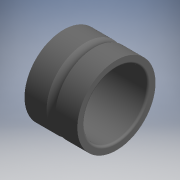
# Autodesk Inventor part: MF63ZZ Inner Ring
Saved by Autodesk Inventor 2017.3 (Build 213256000, 256)
## iProperties
Part Number: MF63ZZ Inner Ring
Material: Generic
Catalog Web Link: www.cadenas.de
Description: shielded_type_zz_zzs_IR-
Vendor: NSK_RB
Document SubType Name: Modeling
Designer: partserver
Manufacturer: NSK_RB
Mass: 0.00900788 g
Surface Area: 0.59285 cm^2
Volume: 0.00900788 cm^3
Density: 1 g/cm^3
Appearance: PSOLRGB-128-128-128
Category: PARTsolutions
Company: NSK_RB
Title: MF63ZZ Inner Ring
Author: Cadenas PARTsolutions
PSOL_IDENT_0: {$CADENAS_DATA\23d-libs\nsk_rb\roller_bearings\deep_groove_bb\exstra_small_miniatur_bb\metric_design
PSOL_IDENT_1: _with_flange\shielded_type_zz_zzs_ir_1.prj},192 {VTYP=3D},{NB=MF63ZZ Inner Ring},{LINA=MF63ZZ Inner
PSOL_IDENT_2: Ring},{NN=shielded_type_zz_zzs_IR},{DATE=10.04.2020 04:57:40},{GEOMDATE=04.01.2008 00:00:00},{VERSIO
PSOL_IDENT_3: N=},{LINEID=120},{WBVAR=},{WBNUMERIC=}  {NB=MF63ZZ Inner Ring},{LINA=MF63ZZ Inner Ring},{KT=DUMMY},{
PSOL_IDENT_4: IDNR=},{STAN=},{ORDER=MF63ZZ},{SD=3.0},{X=3.0},{D=6},{DD=6},{DD1=0.0},{D2=7.2},{DD2=7.2},{B=0.0},{B1=
PSOL_IDENT_5: 2.5},{CC1=0.0},{C2=0.6},{CC2=0.6},{R=0.00},{R1=0.10},{DI1=3.70},{DI2=3.70},{SDE1=4.90},{SDE2=5.40},{
PSOL_IDENT_6: CR1=208},{COR1=74},{CR2=21},{COR2=7.5},{LG=71000},{LO=80000},{DA=0.0},{DB=3.7},{RA=0.00},{RB=0.10},{
PSOL_IDENT_7: MASS=0.33},{SC=1},{N=12}
NB: MF63ZZ Inner Ring
NN: shielded_type_zz_zzs_IR
NBSYN: $ORDER. Inner Ring
LINA: MF63ZZ Inner Ring
CATALOG: NSK Rolling Bearing
ORDER: MF63ZZ
SD: 3
X: 3
D: 6
DD: 6
DD1: 0
D2: 7.2
DD2: 7.2
B: 0
B1: 2.5
CC1: 0
C2: 0.6
CC2: 0.6
R: 0
R1: 0.1
DI1: 3.7
DI2: 3.7
SDE1: 4.9
SDE2: 5.4
CR1: 208
COR1: 74
CR2: 21
COR2: 7.5
LG: 71000
LO: 80000
DA: 0
DB: 3.7
RA: 0
RB: 0.1
MASS: 0.33
SC: 1
SUPPLIER: NSK_RB
ARTICLENO: MF63ZZ Inner Ring
BOMINFO: MF63ZZ Inner Ring
CREATOR: CADENAS GmbH
Autodesk Inventor part; units mm, degrees
sketch "Sketch_1" plane through (0, 0, 0) normal (0, 0, 1) x (1, 0, 0)
  line L0 (2.5, 0) -> (0, 0)
  arc A0 (0, 1.6) -> (0.1, 1.5) centre (0.1, 1.6) ccw
  line L1 (0.1, 1.5) -> (2.4, 1.5)
  arc A1 (2.4, 1.5) -> (2.5, 1.6) centre (2.4, 1.6) ccw
  line L2 (2.5, 1.6) -> (2.5, 1.85)
  line L3 (2.5, 1.85) -> (1.4562, 1.85)
  arc A2 (1.0438, 1.85) -> (1.4562, 1.85) centre (1.25, 2.25) ccw
  line L4 (1.0438, 1.85) -> (0, 1.85)
  line L5 (0, 1.85) -> (0, 1.6)
  constraints: 12 end point, 6 point on circle, 3 centre point
revolve "Revolution1" add sketch "Sketch_1" angle 360 about axis through (2.5, 0, 0) along (1, 0, 0)
ref_plane "ip_st_1_1_XY" through (1.25, 2.25, 0) normal (1, 0, 0) x (0, 0, -1)
ref_plane "ip_st_1_1_YZ" through (1.25, 2.25, 0) normal (0, 0, -1) x (0, 1, 0)
ref_plane "ip_st_1_1_ZX" through (1.25, 2.25, 0) normal (0, 1, 0) x (1, 0, 0)
ref_plane "ip_st_1_10_XY" through (1.25, 0, -2.25) normal (1, 0, 0) x (0, 0, -1)
ref_plane "ip_st_1_10_YZ" through (1.25, 0, -2.25) normal (0, 0, -1) x (0, 1, 0)
ref_plane "ip_st_1_10_ZX" through (1.25, 0, -2.25) normal (0, 1, 0) x (1, 0, 0)
ref_plane "ip_st_1_11_XY" through (1.25, 1.125, -1.9486) normal (1, 0, 0) x (0, 0, -1)
ref_plane "ip_st_1_11_YZ" through (1.25, 1.125, -1.9486) normal (0, 0, -1) x (0, 1, 0)
ref_plane "ip_st_1_11_ZX" through (1.25, 1.125, -1.9486) normal (0, 1, 0) x (1, 0, 0)
ref_plane "ip_st_1_12_XY" through (1.25, 1.9486, -1.125) normal (1, 0, 0) x (0, 0, -1)
ref_plane "ip_st_1_12_YZ" through (1.25, 1.9486, -1.125) normal (0, 0, -1) x (0, 1, 0)
ref_plane "ip_st_1_12_ZX" through (1.25, 1.9486, -1.125) normal (0, 1, 0) x (1, 0, 0)
ref_plane "ip_st_1_2_XY" through (1.25, 1.9486, 1.125) normal (1, 0, 0) x (0, 0, -1)
ref_plane "ip_st_1_2_YZ" through (1.25, 1.9486, 1.125) normal (0, 0, -1) x (0, 1, 0)
ref_plane "ip_st_1_2_ZX" through (1.25, 1.9486, 1.125) normal (0, 1, 0) x (1, 0, 0)
ref_plane "ip_st_1_3_XY" through (1.25, 1.125, 1.9486) normal (1, 0, 0) x (0, 0, -1)
ref_plane "ip_st_1_3_YZ" through (1.25, 1.125, 1.9486) normal (0, 0, -1) x (0, 1, 0)
ref_plane "ip_st_1_3_ZX" through (1.25, 1.125, 1.9486) normal (0, 1, 0) x (1, 0, 0)
ref_plane "ip_st_1_4_XY" through (1.25, 0, 2.25) normal (1, 0, 0) x (0, 0, -1)
ref_plane "ip_st_1_4_YZ" through (1.25, 0, 2.25) normal (0, 0, -1) x (0, 1, 0)
ref_plane "ip_st_1_4_ZX" through (1.25, 0, 2.25) normal (0, 1, 0) x (1, 0, 0)
ref_plane "ip_st_1_5_XY" through (1.25, -1.125, 1.9486) normal (1, 0, 0) x (0, 0, -1)
ref_plane "ip_st_1_5_YZ" through (1.25, -1.125, 1.9486) normal (0, 0, -1) x (0, 1, 0)
ref_plane "ip_st_1_5_ZX" through (1.25, -1.125, 1.9486) normal (0, 1, 0) x (1, 0, 0)
ref_plane "ip_st_1_6_XY" through (1.25, -1.9486, 1.125) normal (1, 0, 0) x (0, 0, -1)
ref_plane "ip_st_1_6_YZ" through (1.25, -1.9486, 1.125) normal (0, 0, -1) x (0, 1, 0)
ref_plane "ip_st_1_6_ZX" through (1.25, -1.9486, 1.125) normal (0, 1, 0) x (1, 0, 0)
ref_plane "ip_st_1_7_XY" through (1.25, -2.25, 0) normal (1, 0, 0) x (0, 0, -1)
ref_plane "ip_st_1_7_YZ" through (1.25, -2.25, 0) normal (0, 0, -1) x (0, 1, 0)
ref_plane "ip_st_1_7_ZX" through (1.25, -2.25, 0) normal (0, 1, 0) x (1, 0, 0)
ref_plane "ip_st_1_8_XY" through (1.25, -1.9486, -1.125) normal (1, 0, 0) x (0, 0, -1)
ref_plane "ip_st_1_8_YZ" through (1.25, -1.9486, -1.125) normal (0, 0, -1) x (0, 1, 0)
ref_plane "ip_st_1_8_ZX" through (1.25, -1.9486, -1.125) normal (0, 1, 0) x (1, 0, 0)
ref_plane "ip_st_1_9_XY" through (1.25, -1.125, -1.9486) normal (1, 0, 0) x (0, 0, -1)
ref_plane "ip_st_1_9_YZ" through (1.25, -1.125, -1.9486) normal (0, 0, -1) x (0, 1, 0)
ref_plane "ip_st_1_9_ZX" through (1.25, -1.125, -1.9486) normal (0, 1, 0) x (1, 0, 0)
ref_plane "ip_st_1a_XY" through (0, 0, 0) normal (1, 0, 0) x (0, 0, -1)
ref_plane "ip_st_1a_YZ" through (0, 0, 0) normal (0, 0, -1) x (0, 1, 0)
ref_plane "ip_st_1a_ZX" through (0, 0, 0) normal (0, 1, 0) x (1, 0, 0)
ref_plane "ip_st_2a_XY" through (0.1562, 0, 0) normal (1, 0, 0) x (0, 0, -1)
ref_plane "ip_st_2a_YZ" through (0.1562, 0, 0) normal (0, 0, -1) x (0, 1, 0)
ref_plane "ip_st_2a_ZX" through (0.1562, 0, 0) normal (0, 1, 0) x (1, 0, 0)
body "Solid1"
